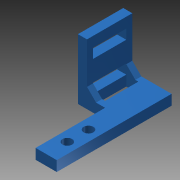
# Autodesk Inventor part: switch bracket v5
Saved by Autodesk Inventor 2013 SP2 (Build 170200200, 200)
## iProperties
Created: 2018-01-15
Part Number: switch bracket v5
Material: Generic
Document SubType Name: Modeling
Designer: hdv
Density: 1 g/cm^3
Author: hdv
Autodesk Inventor part; units mm, degrees
ref_plane "YZ Plane" through (0, 0, 0) normal (1, 0, 0) x (0, 1, 0)
ref_plane "XZ Plane" through (0, 0, 0) normal (0, 1, 0) x (-1, 0, 0)
ref_plane "XY Plane" through (0, 0, 0) normal (0, 0, 1) x (1, 0, 0)
sketch "Sketch1" plane through (0, 0, 0) normal (0, 0, 1) x (1, 0, 0)
  line L0 (0, 0) -> (7, 0)
  line L1 (7, 0) -> (7, 38)
  line L2 (7, 38) -> (0, 38)
  line L3 (0, 38) -> (0, 0)
  circle A0 centre (3.5, 7) radius 1.6
  circle A1 centre (3.5, 14) radius 1.6
  line L4 (0, 38) -> (-9, 38)
  line L5 (-9, 38) -> (-9, 23)
  line L6 (-9, 23) -> (0, 23)
  line L7 (0, 23) -> (0, 38)
  point P0 (3.5, 0)
  dimension "d0" = 7
  dimension "d1" = 38
  dimension "d2" = 3.2
  dimension "d3" = 3.2
  dimension "d4" = 7
  dimension "d5" = 7
  dimension "d7" = 15
  dimension "d8" = 16
  constraints: 16 end point, 4 parallel, 2 centre point, 2 horizontal, 2 perpendicular, 2 vertical alignment, 1 midpoint
  measures "d0" distance of L2.end L1.end
  measures "d1" distance of L1.end L0.end
  measures "d2" diameter of A0
  measures "d3" diameter of A1
  measures "d4" distance of A1.centre A0.centre
  measures "d5" distance from line of A0.centre L0
  measures "d7" distance of L4.end L5.end
  measures "d8" distance between parallel lines of L1 L5
extrude "Extrusion1" add sketch "Sketch1" along normal blind 3.4
sketch "Sketch2" plane through (-9, 23, 0) normal (-1, 0, 0) x (0, 0, 1)
  line L0 (0, 15) -> (0, 0) projected
  line L1 (0, 0) -> (3.4, 0) projected
  line L2 (3.4, 15) -> (3.4, 0) projected
  line L3 (0, 15) -> (3.4, 15) projected
  line L4 (0, 15) -> (20, 15)
  line L5 (20, 15) -> (20, 0)
  line L6 (20, 0) -> (0, 0)
  line L7 (0, 0) -> (0, 15)
  line L8 (3.4, 13) -> (6.6, 13)
  line L9 (6.6, 13) -> (6.6, 2)
  line L10 (6.6, 2) -> (3.4, 2)
  line L11 (3.4, 2) -> (3.4, 13)
  line L12 (13.4, 13) -> (16.6, 13)
  line L13 (16.6, 13) -> (16.6, 2)
  line L14 (16.6, 2) -> (13.4, 2)
  line L15 (13.4, 2) -> (13.4, 13)
  point P0 (0, -23)
  dimension "d11" = 20
  dimension "d12" = 2
  dimension "d13" = 2
  dimension "d14" = 3.2
  dimension "d15" = 3.4
  dimension "d16" = 6.8
  dimension "d17" = 3.2
  constraints: 24 end point, 6 parallel, 3 collinear, 3 horizontal, 3 perpendicular
  measures "d11" distance of L0.start L4.end
  measures "d12" distance between parallel lines of L12 L4
  measures "d13" distance between parallel lines of L6 L14
  measures "d14" distance of L13.end L14.end
  measures "d15" distance between parallel lines of L13 L5
  measures "d16" distance between parallel lines of L9 L15
  measures "d17" distance of L9.end L10.end
extrude "Extrusion2" add sketch "Sketch2" against normal blind 3 contours L4 L5 L6 L2 L10 L9 L8
chamfer "Chamfer1" distance 3 angle 45 2 edges at (-6, 37, 3.4) (-6, 24, 3.4)
sketch "Sketch3" plane through (0, 0, 3.4) normal (0, 0, 1) x (1, 0, 0)
  line L0 (-9, 25) -> (-6, 25) projected
  line L1 (-6, 36) -> (-2, 36)
  line L2 (-2, 36) -> (-2, 25)
  line L3 (-2, 25) -> (-6, 25)
  line L4 (-6, 25) -> (-6, 36)
  dimension "d20" = 4
  constraints: 8 end point, 2 parallel, 1 collinear, 1 horizontal, 1 perpendicular
  measures "d20" distance of L1.start L1.end
extrude "Extrusion3" cut sketch "Sketch3" against normal blind 4
equation "\"d13\" = d12"
equation "\"d17\" = d14"
body "Solid1"
